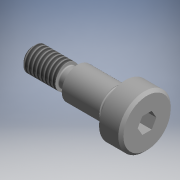
# Autodesk Inventor part: 25-2281_b
Saved by Autodesk Inventor 2017.3 (Build 213256000, 256)
## iProperties
Part Number: 25-2281_b
Material: Generic
Catalog Web Link: www.cadenas.de
Description: 25-2281, 65-2282, 40-2280, 40-2290_b-Roller Wheels
Vendor: 8020
Document SubType Name: Modeling
Designer: partserver
Manufacturer: 8020
Mass: 1.56273 g
Surface Area: 10.5351 cm^2
Volume: 1.56273 cm^3
Density: 1 g/cm^3
Appearance: PSOLRGB-192-192-192
Category: PARTsolutions
Company: 8020
Title: 25-2281_b
Author: Cadenas PARTsolutions
Comments: Roller Wheels
PSOL_IDENT_0: {$CADENAS_DATA\23d-libs\8020\metric\linear_motion\25_2281_bolt.prj},193 {VTYP=3D},{NB=25-2281_b},{LI
PSOL_IDENT_1: NA=25-2281_b},{NN=25-2281, 65-2282, 40-2280, 40-2290_b},{DATE=31.07.2020 09:21:29},{GEOMDATE=22.03.2
PSOL_IDENT_2: 012 00:00:00},{VERSION=},{LINEID=10},{WBVAR=BT,RI},{WBNUMERIC=}  {NB=25-2281_b},{LINA=25-2281_b},{KT=
PSOL_IDENT_3: DUMMY},{PN=25-2281},{NO=1},{MAT=Self-lubricating, fiberglass-reinforced black nylon.},{BT=2},{BT1= '
PSOL_IDENT_4: 2','Permanent Lubricated Bronze Bushing' },{MT=25 Series},{RI=25},{RI1= '25','25 Series','40','40 Se
PSOL_IDENT_5: ries' },{A=37.500},{B=28.000},{C=6.100},{D=12.000},{E=14.000},{F=4.750},{G=8.000},{H=5.500},{J=2.600
PSOL_IDENT_6: 00000},{K=15.900},{L=13.200},{M=8.65000000},{N=M6 x 1.0},{N1=6.0000},{P=1.600},{Q=9.200},{W=.032},{G
PSOL_IDENT_7: 1=10.000},{K1=0.000},{NTP=3382},{WF=4.08400},{T=3.30000}
NB: 25-2281_b
NN: 25-2281, 65-2282, 40-2280, 40-2290_b
NT: Roller Wheels
NBSYN: $PN._b
LINA: 25-2281_b
CATALOG: 80/20
NO: 1
MAT: Self-lubricating, fiberglass-reinforced black nylon.
BT: Permanent Lubricated Bronze Bushing
MT: 25 Series
RI: 25 Series
A: 37.5
B: 28
D: 12
E: 14
F: 4.75
G: 8
H: 5.5
J: 2.6
K: 15.9
L: 13.2
M: 8.65
N: M6 x 1.0
N1: 6
P: 1.6
Q: 9.2
K1: 0
NTP: 3382
WF: 4.084
T: 3.3
SUPPLIER: 8020
ARTICLENO: 25-2281_b
BOMINFO: 25-2281_b
CREATOR: CADENAS GmbH
Autodesk Inventor part; units mm, degrees
ref_plane "YZ Plane" through (0, 0, 0) normal (1, 0, 0) x (0, 1, 0)
ref_plane "XZ Plane" through (0, 0, 0) normal (0, 1, 0) x (-1, 0, 0)
ref_plane "XY Plane" through (0, 0, 0) normal (0, 0, 1) x (1, 0, 0)
sketch "Sketch_1" plane through (0, 0, 0) normal (0, 0, 1) x (1, 0, 0)
  line L0 (23.25, 0) -> (-5.5, 0)
  line L1 (-5.5, 0) -> (-5.5, 5.95)
  line L2 (-5.5, 5.95) -> (-4.85, 6.6)
  line L3 (-4.85, 6.6) -> (0, 6.6)
  line L4 (0, 6.6) -> (0, 3.71)
  line L5 (0, 3.71) -> (2.246, 3.71)
  arc A0 (2.246, 3.71) -> (2.4983, 3.9935) centre (2.246, 3.964) ccw
  line L6 (2.4983, 3.9935) -> (12, 3.9935)
  line L7 (12, 3.9935) -> (12, 2.708)
  arc A1 (12, 2.708) -> (12.508, 2.2) centre (12.508, 2.708) ccw
  line L8 (12.508, 2.2) -> (14.346, 2.2)
  arc A2 (14.346, 2.2) -> (14.6, 2.454) centre (14.346, 2.454) ccw
  line L9 (14.6, 2.454) -> (14.6, 3)
  line L10 (14.6, 3) -> (22.6365, 3)
  line L11 (22.6365, 3) -> (23.25, 2.3865)
  line L12 (23.25, 2.3865) -> (23.25, 0)
  line L13 (23.25, 0) -> (-5.5, 0)
  constraints: 28 end point, 6 point on circle, 3 centre point
revolve "Revolution1" add sketch "Sketch_1" angle 360 about axis through (23.25, 0, 0) along (1, 0, 0)
thread "Thread1" size "M6x1" class "6g" standard "ISO Metric profile" full length
sketch "Sketch_5" plane through (-5.5, 0, 0) normal (1, 0, 0) x (0, 0, -1)
  line L0 (-2.042, -1.1789) -> (0, -2.3579)
  line L1 (0, -2.3579) -> (2.042, -1.1789)
  line L2 (2.042, -1.1789) -> (2.042, 1.1789)
  line L3 (2.042, 1.1789) -> (0, 2.3579)
  line L4 (0, 2.3579) -> (-2.042, 1.1789)
  line L5 (-2.042, 1.1789) -> (-2.042, -1.1789)
  constraints: 12 end point
extrude "Extrusion1" cut sketch "Sketch_5" along normal blind 3.3
ref_plane "bolt_XY" through (0, 0, 0) normal (1, 0, 0) x (0, 0, -1)
ref_plane "bolt_YZ" through (0, 0, 0) normal (0, 0, -1) x (0, 1, 0)
ref_plane "bolt_ZX" through (0, 0, 0) normal (0, 1, 0) x (1, 0, 0)
ref_plane "bolt1_XY" through (15.2, 0, 0) normal (1, 0, 0) x (0, 0, -1)
ref_plane "bolt1_YZ" through (15.2, 0, 0) normal (0, 0, -1) x (0, 1, 0)
ref_plane "bolt1_ZX" through (15.2, 0, 0) normal (0, 1, 0) x (1, 0, 0)
body "Solid1"
